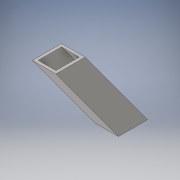
# Autodesk Inventor part: Arm Platform Diagonal strut
Saved by Autodesk Inventor 2016 (Build 200138000, 138)
## iProperties
Created: 2016-02-05
Part Number: Arm Platform Diagonal strut
Material: Generic
Document SubType Name: Modeling
Designer: gus
Density: 1 g/cm^3
Appearance: Default
Author: gus
Autodesk Inventor part; units mm, degrees
ref_plane "YZ Plane" through (0, 0, 0) normal (1, 0, 0) x (0, 1, 0)
ref_plane "XZ Plane" through (0, 0, 0) normal (0, 1, 0) x (-1, 0, 0)
ref_plane "XY Plane" through (0, 0, 0) normal (0, 0, 1) x (1, 0, 0)
sketch "Sketch1" plane through (0, 0, 0) normal (1, 0, 0) x (0, 1, 0)
  line L0 (0, 0) -> (92.075, 67.3887)
  line L1 (92.075, 67.3887) -> (92.075, 98.8649)
  line L2 (92.075, 98.8649) -> (0, 31.4761)
  line L3 (0, 31.4761) -> (0, 0)
  dimension "d0" = 53.8
  dimension "d2" = 25.4
  dimension "d3" = 92.075
  constraints: 8 end point, 2 parallel, 1 vertical
  measures "d0" angle of L0 L3
  measures "d2" distance between parallel lines of L2 L0
  measures "d3" horizontal distance of L0.start L0.end
extrude "Extrusion1" add sketch "Sketch1" along normal blind 25.4
sketch "Sketch3" plane through (0, 0, 0) normal (0, -1, 0) x (1, 0, 0)
  line L0 (22.225, 28.3011) -> (3.175, 28.3011)
  line L1 (3.175, 28.3011) -> (3.175, 3.175)
  line L2 (3.175, 3.175) -> (22.225, 3.175)
  line L3 (22.225, 3.175) -> (22.225, 28.3011)
  line L4 (0, 31.4761) -> (25.4, 31.4761) projected
  line L5 (25.4, 0) -> (25.4, 67.3887) projected
  line L6 (0, 0) -> (25.4, 0) projected
  dimension "d10" = 19.05
  dimension "d12" = 3.175
  dimension "d13" = 3.175
  dimension "d16" = 3.175
  constraints: 8 end point, 2 parallel, 1 horizontal, 1 perpendicular
  measures "d10" distance of L1.end L2.end
  measures "d12" distance between parallel lines of L4 L0
  measures "d13" distance between parallel lines of L5 L3
  measures "d16" distance between parallel lines of L2 L6
sketch3d "3D Sketch1"
  line L0 (25.4, 0, 31.4761) -> (25.4, 92.075, 98.8649)
sweep "Sweep2" cut profiles "Sketch3" path "3D Sketch1"
body "Solid1"
